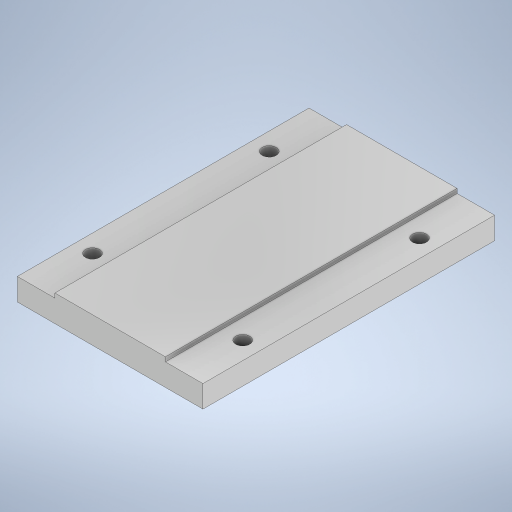
# Autodesk Inventor part: slider_move_gaba
Saved by Autodesk Inventor 2023 (Build 270158000, 158)
## iProperties
Created: 2021-10-23
Part Number: slider_move_gaba
Material: アルミニウム 6061-AHC
Document SubType Name: Modeling
Designer: sky
Density: 2.7 g/cm^3
Appearance: アルミニウム - ダーク
Mass: 41.4427 g
Surface Area: 69.4272 cm^2
Volume: 15.3492 cm^3
Author: sky
Autodesk Inventor part; units mm, degrees
ref_plane "YZ Plane" through (0, 0, 0) normal (1, 0, 0) x (0, 1, 0)
ref_plane "XZ Plane" through (0, 0, 0) normal (0, 1, 0) x (-1, 0, 0)
ref_plane "XY Plane" through (0, 0, 0) normal (0, 0, 1) x (1, 0, 0)
sketch "スケッチ1" plane through (0, 0, 0) normal (0, 1, 0) x (-1, 0, 0)
  line L0 (0, 0) -> (42, 0)
  line L1 (42, 0) -> (42, -66)
  line L2 (42, -66) -> (0, -66)
  line L3 (0, -66) -> (0, 0)
  dimension "d0" = 42
  dimension "d1" = 66
  constraints: 8 end point, 2 parallel, 1 horizontal, 1 perpendicular
  measures "d0" distance of L1.end L2.end
  measures "d1" distance of L0.end L1.end
extrude "押し出し1" add sketch "スケッチ1" along normal blind 5
sketch "スケッチ2" plane through (0, 5, 0) normal (0, 1, 0) x (1, 0, 0)
  line L0 (0, 66) -> (-42, 66) projected
  line L1 (-33.5, 0) -> (-8.5, 0)
  line L2 (-8.5, 0) -> (-8.5, 66)
  line L3 (-8.5, 66) -> (-33.5, 66)
  line L4 (-33.5, 66) -> (-33.5, 0)
  line L5 (-42, 66) -> (-42, 0) projected
  point P0 (0, 0)
  dimension "d4" = 25
  dimension "d5" = 8.5
  constraints: 8 end point, 2 parallel, 1 horizontal, 1 perpendicular, 1 point on line
  measures "d4" distance of L3.end L2.end
  measures "d5" distance between parallel lines of L5 L4
extrude "押し出し2" add sketch "スケッチ2" along normal blind 1
sketch "スケッチ3" plane through (0, 0, 0) normal (0, -1, 0) x (1, 0, 0)
  line L0 (0, 0) -> (0, -66) projected
  line L1 (0, -66) -> (-42, -66) projected
  point P0 (-4, -13)
  point P1 (-4, -53)
  point P2 (-38, -53)
  point P3 (-38, -13)
  dimension "d8" = 40
  dimension "d10" = 4
  dimension "d11" = 13
  measures "d8" distance of point (-4, -53) point (-4, -13)
  measures "d10" distance from line of L0 point (-4, -53)
  measures "d11" distance from line of point (-4, -53) L1
hole "穴1" at (-4, 0, -13) at (-4, 0, -53) at (-38, 0, -53) at (-38, 0, -13) direction (0, 1, 0) diameter 3.2 depth 30 tip angle 118
